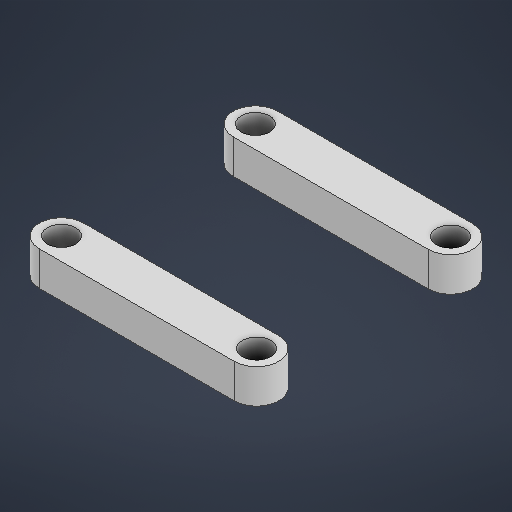
# Autodesk Inventor part: innerBar
Saved by Autodesk Inventor 2026.2 (Build 302298000, 298)
## iProperties
Created: 2026-04-07
Part Number: innerBar
Material: Generic
Document SubType Name: Modeling
Designer: Brian Wang
Density: 1 g/cm^3
Appearance: Default
Author: Brian Wang
Autodesk Inventor part; units mm, degrees
ref_plane "YZ Plane" through (0, 0, 0) normal (1, 0, 0) x (0, 1, 0)
ref_plane "XZ Plane" through (0, 0, 0) normal (0, 1, 0) x (-1, 0, 0)
ref_plane "XY Plane" through (0, 0, 0) normal (0, 0, 1) x (1, 0, 0)
sketch "Sketch1" plane through (0, 0, 0) normal (0, 1, 0) x (-1, 0, 0)
  circle A0 centre (27.2044, 41.0921) radius 2.075
  circle A1 centre (27.2044, 12.7622) radius 2.075
  arc A2 (27.2044, 37.8421) -> (27.2044, 44.3421) centre (27.2044, 41.0921) ccw
  arc A3 (27.2044, 9.5122) -> (27.2044, 16.0122) centre (27.2044, 12.7622) ccw
  circle A4 centre (-1.2956, 41.0921) radius 2.075
  circle A5 centre (-1.2956, 12.7622) radius 2.075
  arc A6 (-1.2956, 44.3421) -> (-1.2956, 37.8421) centre (-1.2956, 41.0921) ccw
  arc A7 (-1.2956, 16.0122) -> (-1.2956, 9.5122) centre (-1.2956, 12.7622) ccw
  line L0 (27.2044, 44.3421) -> (-1.2956, 44.3421)
  line L1 (27.2044, 37.8421) -> (-1.2956, 37.8421)
  line L2 (27.2044, 16.0122) -> (-1.2956, 16.0122)
  line L3 (27.2044, 9.5122) -> (-1.2956, 9.5122)
  point P0 (0, 0)
  dimension "d0" = 4.15
  dimension "d1" = 4.15
  dimension "d2" = 6.5
  dimension "d3" = 4.15
  dimension "d4" = 4.15
  dimension "d5" = 6.5
  dimension "d6" = 28.5
  constraints: 8 centre point, 8 end point, 8 point on circle, 4 coincident, 4 tangent, 2 horizontal alignment, 2 vertical alignment
  measures "d0" diameter of A0
  measures "d1" diameter of A1
  measures "d2" diameter of A2
  measures "d3" diameter of A4
  measures "d4" diameter of A5
  measures "d5" diameter of A6
  measures "d6" distance of A4.centre A0.centre
extrude "Extrusion1" add sketch "Sketch1" along normal blind 5
body "Solid1"
